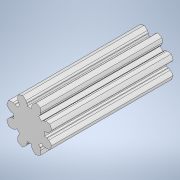
# Autodesk Inventor part: ぴにょん歯数7
Saved by Autodesk Inventor 2022.2 (Build 262287030, 287C)
## iProperties
Created: 2022-02-22
Part Number: ぴにょん歯数7
Material: Aluminum 2014-T6
Document SubType Name: Modeling
Designer: acps
Density: 2.78927 g/cm^3
Appearance: Satin
Author: acps
Autodesk Inventor part; units mm, degrees
ref_plane "YZ Plane" through (0, 0, 0) normal (1, 0, 0) x (0, 1, 0)
ref_plane "XZ Plane" through (0, 0, 0) normal (0, 1, 0) x (-1, 0, 0)
ref_plane "XY Plane" through (0, 0, 0) normal (0, 0, 1) x (1, 0, 0)
sketch "Sketch1" plane through (0, 0, 0) normal (0, 0, 1) x (1, 0, 0)
  arc A0 (0.2626, 1.917) -> (0.2462, 1.8632) centre (0.4994, 1.8157) ccw
  arc A1 (0.3627, 2.0876) -> (0.2626, 1.917) centre (0.9307, 1.6395) ccw
  arc A2 (0.7114, 2.3967) -> (0.3627, 2.0876) centre (1.3933, 1.2761) ccw
  arc A3 (-1.1698, 1.5411) -> (-1.1434, 1.4916) centre (-0.9308, 1.637) ccw
  arc A4 (-1.2197, 1.7326) -> (-1.1698, 1.5411) centre (-0.5012, 1.8175) ccw
  arc A5 (-1.1917, 2.1977) -> (-1.2197, 1.7326) centre (0.0829, 1.8876) ccw
  arc A6 (-1.917, 0.2626) -> (-1.8632, 0.2462) centre (-1.8157, 0.4994) ccw
  arc A7 (-2.0876, 0.3627) -> (-1.917, 0.2626) centre (-1.6395, 0.9307) ccw
  arc A8 (-2.3967, 0.7114) -> (-2.0876, 0.3627) centre (-1.2761, 1.3933) ccw
  arc A9 (-1.5411, -1.1698) -> (-1.4916, -1.1434) centre (-1.637, -0.9308) ccw
  arc A10 (-1.7326, -1.2197) -> (-1.5411, -1.1698) centre (-1.8175, -0.5012) ccw
  arc A11 (-2.1977, -1.1917) -> (-1.7326, -1.2197) centre (-1.8876, 0.0829) ccw
  arc A12 (-0.2626, -1.917) -> (-0.2462, -1.8632) centre (-0.4994, -1.8157) ccw
  arc A13 (-0.3627, -2.0876) -> (-0.2626, -1.917) centre (-0.9307, -1.6395) ccw
  arc A14 (-0.7114, -2.3967) -> (-0.3627, -2.0876) centre (-1.3933, -1.2761) ccw
  arc A15 (1.1698, -1.5411) -> (1.1434, -1.4916) centre (0.9308, -1.637) ccw
  arc A16 (1.2197, -1.7326) -> (1.1698, -1.5411) centre (0.5012, -1.8175) ccw
  arc A17 (1.1917, -2.1977) -> (1.2197, -1.7326) centre (-0.0829, -1.8876) ccw
  arc A18 (1.917, -0.2626) -> (1.8632, -0.2462) centre (1.8157, -0.4994) ccw
  arc A19 (2.0876, -0.3627) -> (1.917, -0.2626) centre (1.6395, -0.9307) ccw
  arc A20 (2.3967, -0.7114) -> (2.0876, -0.3627) centre (1.2761, -1.3933) ccw
  arc A21 (1.5411, 1.1698) -> (1.4916, 1.1434) centre (1.637, 0.9308) ccw
  arc A22 (1.7326, 1.2197) -> (1.5411, 1.1698) centre (1.8175, 0.5012) ccw
  arc A23 (2.1977, 1.1917) -> (1.7326, 1.2197) centre (1.8876, -0.0829) ccw
  arc A24 (-0.2462, 1.8632) -> (-0.2626, 1.917) centre (-0.4994, 1.8157) ccw
  arc A25 (-0.2626, 1.917) -> (-0.3627, 2.0876) centre (-0.9307, 1.6395) ccw
  arc A26 (-0.3627, 2.0876) -> (-0.7114, 2.3967) centre (-1.3933, 1.2761) ccw
  arc A27 (-1.4916, 1.1434) -> (-1.5411, 1.1698) centre (-1.637, 0.9308) ccw
  arc A28 (-1.5411, 1.1698) -> (-1.7326, 1.2197) centre (-1.8175, 0.5012) ccw
  arc A29 (-1.7326, 1.2197) -> (-2.1977, 1.1917) centre (-1.8876, -0.0829) ccw
  arc A30 (-1.8632, -0.2462) -> (-1.917, -0.2626) centre (-1.8157, -0.4994) ccw
  arc A31 (-1.917, -0.2626) -> (-2.0876, -0.3627) centre (-1.6395, -0.9307) ccw
  arc A32 (-2.0876, -0.3627) -> (-2.3967, -0.7114) centre (-1.2761, -1.3933) ccw
  arc A33 (-1.1434, -1.4916) -> (-1.1698, -1.5411) centre (-0.9308, -1.637) ccw
  arc A34 (-1.1698, -1.5411) -> (-1.2197, -1.7326) centre (-0.5012, -1.8175) ccw
  arc A35 (-1.2197, -1.7326) -> (-1.1917, -2.1977) centre (0.0829, -1.8876) ccw
  arc A36 (0.2462, -1.8632) -> (0.2626, -1.917) centre (0.4994, -1.8157) ccw
  arc A37 (0.2626, -1.917) -> (0.3627, -2.0876) centre (0.9307, -1.6395) ccw
  arc A38 (0.3627, -2.0876) -> (0.7114, -2.3967) centre (1.3933, -1.2761) ccw
  arc A39 (1.4916, -1.1434) -> (1.5411, -1.1698) centre (1.637, -0.9308) ccw
  arc A40 (1.5411, -1.1698) -> (1.7326, -1.2197) centre (1.8175, -0.5012) ccw
  arc A41 (1.7326, -1.2197) -> (2.1977, -1.1917) centre (1.8876, 0.0829) ccw
  arc A42 (1.8632, 0.2462) -> (1.917, 0.2626) centre (1.8157, 0.4994) ccw
  arc A43 (1.917, 0.2626) -> (2.0876, 0.3627) centre (1.6395, 0.9307) ccw
  arc A44 (2.0876, 0.3627) -> (2.3967, 0.7114) centre (1.2761, 1.3933) ccw
  arc A45 (1.1434, 1.4916) -> (1.1698, 1.5411) centre (0.9308, 1.637) ccw
  arc A46 (1.1698, 1.5411) -> (1.2197, 1.7326) centre (0.5012, 1.8175) ccw
  arc A47 (1.2197, 1.7326) -> (1.1917, 2.1977) centre (-0.0829, 1.8876) ccw
  arc A48 (0.2162, 1.6358) -> (-0.2162, 1.6358) centre (0, 0) ccw
  arc A49 (-1.0038, 1.3095) -> (-1.3095, 1.0038) centre (0, 0) ccw
  arc A50 (-1.6358, 0.2162) -> (-1.6358, -0.2162) centre (0, 0) ccw
  arc A51 (-1.3095, -1.0038) -> (-1.0038, -1.3095) centre (0, 0) ccw
  arc A52 (-0.2162, -1.6358) -> (0.2162, -1.6358) centre (0, 0) ccw
  arc A53 (1.0038, -1.3095) -> (1.3095, -1.0038) centre (0, 0) ccw
  arc A54 (1.6358, -0.2162) -> (1.6358, 0.2162) centre (0, 0) ccw
  arc A55 (1.3095, 1.0038) -> (1.0038, 1.3095) centre (0, 0) ccw
  arc A56 (-0.7114, 2.3967) -> (-1.1917, 2.1977) centre (0, 0) ccw
  arc A57 (-2.1977, 1.1917) -> (-2.3967, 0.7114) centre (0, 0) ccw
  arc A58 (-2.3967, -0.7114) -> (-2.1977, -1.1917) centre (0, 0) ccw
  arc A59 (-1.1917, -2.1977) -> (-0.7114, -2.3967) centre (0, 0) ccw
  arc A60 (0.7114, -2.3967) -> (1.1917, -2.1977) centre (0, 0) ccw
  arc A61 (2.1977, -1.1917) -> (2.3967, -0.7114) centre (0, 0) ccw
  arc A62 (2.3967, 0.7114) -> (2.1977, 1.1917) centre (0, 0) ccw
  arc A63 (1.1917, 2.1977) -> (0.7114, 2.3967) centre (0, 0) ccw
  line L0 (0.2162, 1.6358) -> (0.2462, 1.8632)
  line L1 (-1.0038, 1.3095) -> (-1.1434, 1.4916)
  line L2 (-1.6358, 0.2162) -> (-1.8632, 0.2462)
  line L3 (-1.3095, -1.0038) -> (-1.4916, -1.1434)
  line L4 (-0.2162, -1.6358) -> (-0.2462, -1.8632)
  line L5 (1.0038, -1.3095) -> (1.1434, -1.4916)
  line L6 (1.6358, -0.2162) -> (1.8632, -0.2462)
  line L7 (1.3095, 1.0038) -> (1.4916, 1.1434)
  line L8 (-0.2162, 1.6358) -> (-0.2462, 1.8632)
  line L9 (-1.3095, 1.0038) -> (-1.4916, 1.1434)
  line L10 (-1.6358, -0.2162) -> (-1.8632, -0.2462)
  line L11 (-1.0038, -1.3095) -> (-1.1434, -1.4916)
  line L12 (0.2162, -1.6358) -> (0.2462, -1.8632)
  line L13 (1.3095, -1.0038) -> (1.4916, -1.1434)
  line L14 (1.6358, 0.2162) -> (1.8632, 0.2462)
  line L15 (1.0038, 1.3095) -> (1.1434, 1.4916)
  point P0 (0, 0)
  constraints: 128 point on circle, 64 centre point, 32 end point
extrude "Extrusion1" add sketch "Sketch1" against normal blind 13
body "Solid1"
